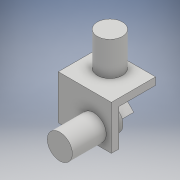
# Autodesk Inventor part: galvos
Saved by Autodesk Inventor 2018 (Build 220112000, 112)
## iProperties
Created: 2018-02-18
Part Number: galvos
Material: Generic
Document SubType Name: Modeling
Designer: gaffo
Density: 1 g/cm^3
Appearance: Default
Author: gaffo
Autodesk Inventor part; units mm, degrees
ref_plane "YZ Plane" through (0, 0, 0) normal (1, 0, 0) x (0, 1, 0)
ref_plane "XZ Plane" through (0, 0, 0) normal (0, 1, 0) x (-1, 0, 0)
ref_plane "XY Plane" through (0, 0, 0) normal (0, 0, 1) x (1, 0, 0)
sketch "Sketch1" plane through (0, 0, 0) normal (0, 1, 0) x (-1, 0, 0)
  line L0 (18, 15) -> (-18, 15)
  line L1 (-18, 15) -> (-18, -15)
  line L2 (-18, -15) -> (18, -15)
  line L3 (18, -15) -> (18, 15)
  point P0 (0, 0)
  point P1 (18, 0)
  point P2 (0, 15)
  dimension "d0" = 36
  dimension "d1" = 30
  constraints: 8 end point, 2 midpoint, 2 parallel, 1 horizontal, 1 horizontal alignment, 1 perpendicular, 1 vertical alignment
  measures "d0" distance between parallel lines of L1 L3
  measures "d1" distance between parallel lines of L2 L0
extrude "Extrusion1" add sketch "Sketch1" along normal blind 5
sketch "Sketch2" plane through (0, 5, 0) normal (0, 1, 0) x (1, 0, 0)
  line L0 (-18, -15) -> (18, -15) projected
  line L1 (-18, -15) -> (18, -15)
  line L2 (18, -15) -> (18, -10)
  line L3 (18, -10) -> (-18, -10)
  line L4 (-18, -10) -> (-18, -15)
  point P0 (0, 0)
  dimension "d4" = 5
  constraints: 8 end point, 2 parallel, 1 horizontal, 1 perpendicular
  measures "d4" distance between parallel lines of L3 L0
extrude "Extrusion2" add sketch "Sketch2" along normal blind 25
sketch "Sketch3" plane through (0, 0, 0) normal (0, -1, 0) x (1, 0, 0)
  circle A0 centre (6, -5.5) radius 8.5
  line L0 (-18, 15) -> (18, 15) projected
  line L1 (18, 15) -> (18, -15) projected
  point P0 (0, 0)
  dimension "dGalvo" = 17
  dimension "d8" = 20.5
  dimension "d9" = 3.5
  constraints: 1 centre point
  measures "dGalvo" diameter of A0
  measures "d8" distance from line of A0.centre L0
  measures "d9" distance edge to line of A0 L1
extrude "Extrusion3" add sketch "Sketch3" along normal blind 23
sketch "Sketch4" plane through (-18, 0, 15) normal (0, 0, 1) x (1, 0, 0)
  circle A0 centre (15.5, 19.5) radius 8.5
  line L0 (0, 30) -> (36, 30) projected
  line L1 (0, 0) -> (0, 30) projected
  point P0 (18, 0)
  dimension "d12" = 17
  dimension "d13" = 2
  dimension "d14" = 15.5
  constraints: 1 centre point
  measures "d12" diameter of A0
  measures "d13" distance edge to line of A0 L0
  measures "d14" distance from line of A0.centre L1
extrude "Extrusion4" add sketch "Sketch4" along normal blind 23
sketch "Sketch5" plane through (18, 5, 10) normal (0, 0, -1) x (-1, 0, 0)
  circle A0 centre (20.5, 14.5) radius 8.5 projected
  point P0 (18, -5)
extrude "Extrusion5" add sketch "Sketch5" along normal blind 6.38
sketch "Sketch6" plane through (0, 5, 0) normal (0, 1, 0) x (1, 0, 0)
  circle A0 centre (6, 5.5) radius 8.5 projected
  point P0 (0, 0)
extrude "Extrusion6" add sketch "Sketch6" along normal blind 6.38
sketch "Sketch7" plane through (6, 11.38, -5.5) normal (0, 1, 0) x (1, 0, 0)
  line L0 (-2.1213, -2.8284) -> (2.8284, 2.1213)
  line L1 (2.8284, 2.1213) -> (2.1213, 2.8284)
  line L2 (2.1213, 2.8284) -> (-2.8284, -2.1213)
  line L3 (-2.8284, -2.1213) -> (-2.1213, -2.8284)
  circle A0 centre (0, 0) radius 8.5 projected
  point P0 (-6, -5.5)
  point P1 (-2.4749, -2.4749)
  point P2 (0.3536, -0.3536)
  dimension "lenMirror" = 7
  dimension "thicknessMirror" = 1
  constraints: 8 end point, 2 midpoint, 2 parallel, 1 perpendicular
  measures "lenMirror" distance of L2.end L1.end
  measures "thicknessMirror" distance of L1.end L0.end
extrude "Extrusion7" add sketch "Sketch7" along normal blind 13 contours L3 L2 L1 L0
sketch "Sketch8" plane through (-2.5, 19.5, 3.62) normal (0, 0, -1) x (-1, 0, 0)
  circle A0 centre (0, 0) radius 8.5 projected
  line L0 (2.1213, 2.8284) -> (-2.8284, -2.1213)
  line L1 (-2.8284, -2.1213) -> (-2.1213, -2.8284)
  line L2 (-2.1213, -2.8284) -> (2.8284, 2.1213)
  line L3 (2.8284, 2.1213) -> (2.1213, 2.8284)
  point P0 (-2.5, -19.5)
  point P1 (2.4749, 2.4749)
  point P2 (-0.3536, 0.3536)
  dimension "d25" = 7
  dimension "d26" = 1
  constraints: 8 end point, 2 midpoint, 2 parallel, 1 perpendicular
  measures "d25" distance between parallel lines of L1 L3
  measures "d26" distance between parallel lines of L0 L2
extrude "Extrusion8" add sketch "Sketch8" along normal blind 13 contours L3 L2 L1 L0
equation "\"d12\" = dGalvo"
equation "\"d15\" = depthGalvo"
equation "\"d19\" = depthGalvoHead"
equation "\"d25\" = lenMirror"
equation "\"d26\" = thicknessMirror"
equation "\"d27\" = depthMirror"
equation "\"depthGalvo\" = 23"
equation "\"depthGalvoHead\" = 6.38"
equation "\"depthMirror\" = 13"
body "Solid1"
